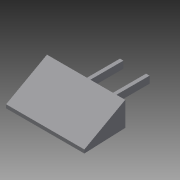
# Autodesk Inventor part: Prow
Saved by Autodesk Inventor 2015 (Build 190159000, 159)
## iProperties
Created: 2016-01-19
Part Number: Prow
Material: Generic
Document SubType Name: Modeling
Designer: sethbattis
Density: 1 g/cm^3
Appearance: Default
Author: sethbattis
Autodesk Inventor part; units mm, degrees
ref_plane "YZ Plane" through (0, 0, 0) normal (1, 0, 0) x (0, 1, 0)
ref_plane "XZ Plane" through (0, 0, 0) normal (0, 1, 0) x (-1, 0, 0)
ref_plane "XY Plane" through (0, 0, 0) normal (0, 0, 1) x (1, 0, 0)
sketch "Sketch1" plane through (0, 0, 0) normal (1, 0, 0) x (0, 1, 0)
  line L0 (-127, 381) -> (-127, -77.6639) construction
  line L1 (0, -661.9789) -> (0, 573.9217) construction
  line L2 (-325.9714, 0) -> (482.0293, 0) construction
  line L3 (76.331, 381) -> (-127, 381) construction
  line L4 (177.8, 0) -> (50.8, 0) construction
  line L5 (50.8, 0) -> (50.8, 50.8) construction
  line L6 (82.55, 82.55) -> (146.05, 82.55) construction
  line L7 (177.8, 50.8) -> (177.8, 0) construction
  arc A0 (177.8, 50.8) -> (146.05, 82.55) centre (146.05, 50.8) ccw construction
  arc A1 (82.55, 82.55) -> (50.8, 50.8) centre (82.55, 50.8) ccw construction
  line L8 (0, 381) -> (-25.4, 381)
  line L9 (-25.4, 381) -> (-12.7354, 82.55)
  line L10 (-12.7354, 82.55) -> (76.0809, 82.55)
  line L11 (164.7876, 82.55) -> (0, 381)
  line L12 (50.8, -196.85) -> (50.8, 0) construction
  line L13 (50.8, -196.85) -> (0, -196.85) construction
  line L14 (39.8671, 0) -> (0, -196.85) construction
  line L15 (78.029, -196.85) -> (147.2733, 83.2908) construction
  line L16 (147.2733, 83.2908) -> (233.3883, 62.0051) construction
  line L17 (233.3883, 62.0051) -> (145.0014, 391.2696) construction
  line L18 (145.0014, 391.2696) -> (120.3435, 397.3645) construction
  line L19 (120.3435, 397.3645) -> (61.0518, 104.6027) construction
  line L20 (61.0518, 104.6027) -> (147.2733, 83.2908) construction
  line L21 (0, -196.85) -> (151.6648, -196.85) construction
  circle A2 centre (78.029, -196.85) radius 288.5717 construction
  line L22 (164.7876, 82.55) -> (76.0809, 82.55)
  point P0 (0, 0)
  point P1 (50.8, 82.55)
  point P2 (177.8, 82.55)
  dimension "d43" = 577.1434
  dimension "d2" = 127
  dimension "d3" = 381
  dimension "d4" = 127
  dimension "d6" = 304.8
  dimension "d7" = 31.75
  dimension "d8" = 25.4
  dimension "d36" = 196.85
  dimension "d37" = 11.449
  dimension "d38" = 61.095
  dimension "d41" = 61.09
  dimension "d42" = 82.55
  constraints: 42 end point, 13 point on line, 6 tangent, 5 collinear, 4 horizontal, 4 perpendicular, 4 point on circle, 3 equal length, 3 parallel, 2 centre point, 1 coincident, 1 equal radius, 1 vertical, 4 other
  measures "d2" distance between parallel lines of L0 L1
  measures "d3" distance between parallel lines of L3 L2
  measures "d4" distance of point (50.8, 82.55) point (177.8, 82.55)
  measures "d6" distance between parallel lines of L0 L7
  measures "d7" radius of A0
  measures "d8" distance of L8.start L8.end
  measures "d36" distance of L12.start L12.end
  measures "d37" angle of L1 L14
  measures "d38" angle of L10 L11
  measures "d41" angle of L16 L17
  measures "d42" distance between parallel lines of L2 L6
extrude "Extrusion1" add sketch "Sketch1" along normal blind 571.5
sketch "Sketch2" plane through (0, -12.7354, 82.55) normal (0, 0, -1) x (-1, 0, 0)
  line L0 (0, 0) -> (0, 177.523) construction
  line L1 (0, 177.523) -> (-571.5, 177.523) construction
  line L2 (-571.5, 0) -> (-571.5, 177.523) construction
  line L3 (0, 0) -> (-571.5, 0) construction
  line L4 (-393.7, 63.5354) -> (-368.3, 63.5354)
  line L5 (-368.3, 63.5354) -> (-368.3, 12.7354)
  line L6 (-368.3, 12.7354) -> (-393.7, 12.7354)
  line L7 (-393.7, 12.7354) -> (-393.7, 63.5354)
  line L8 (0, 12.7354) -> (-571.5, 12.7354) projected
  line L9 (-203.2, 63.5354) -> (-177.8, 63.5354)
  line L10 (-177.8, 63.5354) -> (-177.8, 12.7354)
  line L11 (-177.8, 12.7354) -> (-203.2, 12.7354)
  line L12 (-203.2, 12.7354) -> (-203.2, 63.5354)
  line L13 (0, 177.523) -> (-571.5, 177.523) construction
  line L14 (-285.75, 177.523) -> (-285.75, 0) construction
  dimension "d29" = 25.4
  dimension "d30" = 50.8
  dimension "d31" = 215.9
  constraints: 18 end point, 4 parallel, 2 equal length, 2 horizontal, 2 midpoint, 2 perpendicular, 2 point on line, 1 other
  measures "d29" distance of L5.end L6.end
  measures "d30" distance of L4.end L5.end
  measures "d31" distance between parallel lines of L10 L7
extrude "Extrusion2" add sketch "Sketch2" along normal blind 355.6
body "Solid1"
